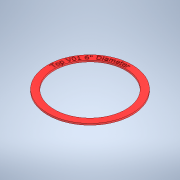
# Autodesk Inventor part: supportRingsForLargeCap
Saved by Autodesk Inventor 2021.1 (Build 251245010, 245A)
## iProperties
Created: 2020-09-25
Part Number: supportRingsForLargeCap
Material: PC/ABS Plastic
Document SubType Name: Modeling
Designer: robst
Density: 0.357273 g/cm^3
Appearance: Light Red
Author: robst
Autodesk Inventor part; units mm, degrees
ref_plane "YZ Plane" through (0, 0, 0) normal (1, 0, 0) x (0, 1, 0)
ref_plane "XZ Plane" through (0, 0, 0) normal (0, 1, 0) x (-1, 0, 0)
ref_plane "XY Plane" through (0, 0, 0) normal (0, 0, 1) x (1, 0, 0)
sketch "Sketch6" plane through (0, 0, 0) normal (0, 0, 1) x (1, 0, 0)
  line L0 (69.85, 0) -> (82.55, 0)
  line L1 (82.55, 0) -> (82.55, 3.175)
  line L2 (82.55, 3.175) -> (69.85, 3.175)
  line L3 (69.85, 3.175) -> (69.85, 0)
  line L4 (0, -0.635) -> (0, 3.81) projected
  point P0 (0, 0)
  dimension "d25" = 12.7
  dimension "d26" = 3.175
  dimension "d27" = 69.85
  constraints: 8 end point, 2 parallel, 1 horizontal, 1 perpendicular
  measures "d25" distance between parallel lines of L1 L3
  measures "d26" distance between parallel lines of L2 L0
  measures "d27" distance of L0.start point (0, 0)
revolve "Revolution3" add sketch "Sketch6" angle 360 about axis through (0, -10, 0) along (0, 1, 0)
sketch "Sketch7" plane through (0, 3.175, 0) normal (0, 1, 0) x (1, 0, 0)
  circle A0 centre (0, 0) radius 76.2 construction
  line L0 (-71.6959, 2.9717) -> (-79.5244, 3.3615)
  line L1 (-79.5244, 3.3615) -> (-79.6728, 0.3827)
  line L2 (-79.6728, 0.3827) -> (-80.7233, 0.435)
  line L3 (-80.7233, 0.435) -> (-80.3678, 7.5727)
  line L4 (-80.3678, 7.5727) -> (-79.3173, 7.5204)
  line L5 (-79.3173, 7.5204) -> (-79.4657, 4.5415)
  line L6 (-79.4657, 4.5415) -> (-71.6372, 4.1517)
  line L7 (-71.6372, 4.1517) -> (-71.6959, 2.9717)
  spline S0 degree 2 poles (-73.8622, 13.8506) (-72.1943, 13.6058) (-70.612, 11.7353) (-70.8087, 10.3953) knots 0 0 0 1 2 2 2
  spline S1 degree 2 poles (-70.8087, 10.3953) (-71.0106, 9.0196) (-73.1164, 7.7194) (-74.7273, 7.9559) knots 0 0 0 1 2 2 2
  spline S2 degree 2 poles (-74.7273, 7.9559) (-76.381, 8.1985) (-77.9743, 10.0925) (-77.7798, 11.4183) knots 0 0 0 1 2 2 2
  spline S3 degree 2 poles (-77.7798, 11.4183) (-77.5831, 12.7583) (-75.523, 14.0943) (-73.8622, 13.8506) knots 0 0 0 1 2 2 2
  spline S4 degree 2 poles (-74.0306, 12.703) (-75.3136, 12.8913) (-76.6981, 12.1406) (-76.8246, 11.2781) knots 0 0 0 1 2 2 2
  spline S5 degree 2 poles (-76.8246, 11.2781) (-76.9512, 10.4157) (-75.8419, 9.2917) (-74.5589, 9.1034) knots 0 0 0 1 2 2 2
  spline S6 degree 2 poles (-74.5589, 9.1034) (-73.3115, 8.9204) (-71.8904, 9.673) (-71.7638, 10.5354) knots 0 0 0 1 2 2 2
  spline S7 degree 2 poles (-71.7638, 10.5354) (-71.6383, 11.3908) (-72.7619, 12.5168) (-74.0306, 12.703) knots 0 0 0 1 2 2 2
  spline S8 degree 2 poles (-72.4154, 20.7565) (-70.7915, 20.3609) (-69.2505, 18.3468) (-69.5387, 17.1639) knots 0 0 0 1 2 2 2
  spline S9 degree 2 poles (-69.5387, 17.1639) (-69.6564, 16.6809) (-70.0611, 15.9935) (-70.3859, 15.6648) knots 0 0 0 1 2 2 2
  line L8 (-70.3859, 15.6648) -> (-67.6701, 15.0032)
  line L9 (-67.6701, 15.0032) -> (-67.9361, 13.9113)
  line L10 (-67.9361, 13.9113) -> (-76.8045, 16.0718)
  line L11 (-76.8045, 16.0718) -> (-76.5385, 17.1638)
  line L12 (-76.5385, 17.1638) -> (-75.8595, 16.9983)
  spline S10 degree 2 poles (-75.8595, 16.9983) (-76.1316, 17.4947) (-76.3794, 18.608) (-76.2379, 19.1889) knots 0 0 0 1 2 2 2
  spline S11 degree 2 poles (-76.2379, 19.1889) (-75.9667, 20.3019) (-73.8993, 21.118) (-72.4154, 20.7565) knots 0 0 0 1 2 2 2
  spline S12 degree 2 poles (-72.564, 19.5989) (-73.6769, 19.8701) (-75.074, 19.4615) (-75.2667, 18.6706) knots 0 0 0 1 2 2 2
  spline S13 degree 2 poles (-75.2667, 18.6706) (-75.3793, 18.2086) (-75.1778, 17.2401) (-74.9496, 16.7767) knots 0 0 0 1 2 2 2
  line L13 (-74.9496, 16.7767) -> (-71.2678, 15.8797)
  spline S14 degree 2 poles (-71.2678, 15.8797) (-70.9608, 16.2572) (-70.6585, 16.8287) (-70.563, 17.2206) knots 0 0 0 1 2 2 2
  spline S15 degree 2 poles (-70.563, 17.2206) (-70.3567, 18.0676) (-71.3741, 19.309) (-72.564, 19.5989) knots 0 0 0 1 2 2 2
  line L14 (-73.177, 34.0889) -> (-66.1232, 27.8719)
  line L15 (-66.1232, 27.8719) -> (-66.6089, 26.6929)
  line L16 (-66.6089, 26.6929) -> (-75.995, 27.2478)
  line L17 (-75.995, 27.2478) -> (-75.5121, 28.4201)
  line L18 (-75.5121, 28.4201) -> (-67.7459, 27.8859)
  line L19 (-67.7459, 27.8859) -> (-73.6353, 32.9764)
  line L20 (-73.6353, 32.9764) -> (-73.177, 34.0889)
  spline S16 degree 2 poles (-65.9446, 38.2865) (-63.8327, 37.1636) (-62.5072, 34.884) (-63.1871, 33.6055) knots 0 0 0 1 2 2 2
  spline S17 degree 2 poles (-63.1871, 33.6055) (-63.877, 32.3079) (-66.5394, 32.1651) (-68.6067, 33.2643) knots 0 0 0 1 2 2 2
  spline S18 degree 2 poles (-68.6067, 33.2643) (-70.7313, 34.3939) (-72.0441, 36.6667) (-71.3609, 37.9516) knots 0 0 0 1 2 2 2
  spline S19 degree 2 poles (-71.3609, 37.9516) (-70.6743, 39.2429) (-67.9928, 39.3755) (-65.9446, 38.2865) knots 0 0 0 1 2 2 2
  spline S20 degree 2 poles (-64.2699, 35.6662) (-64.5767, 36.0252) (-65.7049, 36.7883) (-66.5128, 37.2178) knots 0 0 0 1 2 2 2
  spline S21 degree 2 poles (-66.5128, 37.2178) (-67.3206, 37.6474) (-68.5777, 38.1526) (-69.063, 38.2067) knots 0 0 0 1 2 2 2
  spline S22 degree 2 poles (-69.063, 38.2067) (-69.5483, 38.2607) (-70.256, 37.9272) (-70.4894, 37.4883) knots 0 0 0 1 2 2 2
  spline S23 degree 2 poles (-70.4894, 37.4883) (-70.7228, 37.0493) (-70.6103, 36.2634) (-70.2848, 35.8782) knots 0 0 0 1 2 2 2
  spline S24 degree 2 poles (-70.2848, 35.8782) (-69.9686, 35.5061) (-68.8082, 34.7422) (-68.0385, 34.3329) knots 0 0 0 1 2 2 2
  spline S25 degree 2 poles (-68.0385, 34.3329) (-67.2116, 33.8932) (-66.0507, 33.4065) (-65.5302, 33.3419) knots 0 0 0 1 2 2 2
  spline S26 degree 2 poles (-65.5302, 33.3419) (-65.0419, 33.2781) (-64.302, 33.6109) (-64.0585, 34.0689) knots 0 0 0 1 2 2 2
  spline S27 degree 2 poles (-64.0585, 34.0689) (-63.8285, 34.5014) (-63.941, 35.2874) (-64.2699, 35.6662) knots 0 0 0 1 2 2 2
  line L21 (-58.6672, 41.3818) -> (-61.0498, 37.7579)
  line L22 (-61.0498, 37.7579) -> (-61.8083, 38.2566)
  line L23 (-61.8083, 38.2566) -> (-60.9217, 39.605)
  line L24 (-60.9217, 39.605) -> (-65.9001, 42.878)
  line L25 (-65.9001, 42.878) -> (-66.7866, 41.5296)
  line L26 (-66.7866, 41.5296) -> (-67.4668, 41.9768)
  spline S28 degree 2 poles (-67.4668, 41.9768) (-66.9642, 42.7413) (-66.9227, 43.7486) (-67.493, 44.1926) knots 0 0 0 1 2 2 2
  line L27 (-67.493, 44.1926) -> (-66.9864, 44.9631)
  line L28 (-66.9864, 44.9631) -> (-60.2925, 40.5621)
  line L29 (-60.2925, 40.5621) -> (-59.4257, 41.8804)
  line L30 (-59.4257, 41.8804) -> (-58.6672, 41.3818)
  spline S29 degree 2 poles (-53.7813, 51.8344) (-53.2703, 51.3792) (-52.7061, 50.2688) (-52.6695, 49.7249) knots 0 0 0 1 2 2 2
  spline S30 degree 2 poles (-52.6695, 49.7249) (-52.6265, 49.1559) (-52.9704, 48.1308) (-53.3681, 47.6843) knots 0 0 0 1 2 2 2
  spline S31 degree 2 poles (-53.3681, 47.6843) (-53.7658, 47.2378) (-54.7236, 46.7692) (-55.274, 46.7578) knots 0 0 0 1 2 2 2
  spline S32 degree 2 poles (-55.274, 46.7578) (-55.9411, 46.7346) (-57.4965, 47.4254) (-58.3787, 48.2113) knots 0 0 0 1 2 2 2
  spline S33 degree 2 poles (-58.3787, 48.2113) (-59.2448, 48.9828) (-60.3218, 50.579) (-60.5076, 51.4102) knots 0 0 0 1 2 2 2
  spline S34 degree 2 poles (-60.5076, 51.4102) (-60.6922, 52.221) (-60.2411, 53.8646) (-59.5751, 54.6123) knots 0 0 0 1 2 2 2
  spline S35 degree 2 poles (-59.5751, 54.6123) (-59.3786, 54.8329) (-58.9905, 55.1819) (-58.8128, 55.284) knots 0 0 0 1 2 2 2
  line L31 (-58.8128, 55.284) -> (-57.9574, 54.5221)
  line L32 (-57.9574, 54.5221) -> (-57.991, 54.4844)
  spline S36 degree 2 poles (-57.991, 54.4844) (-58.1657, 54.4182) (-58.6812, 54.067) (-58.9112, 53.8088) knots 0 0 0 1 2 2 2
  spline S37 degree 2 poles (-58.9112, 53.8088) (-59.6492, 52.9803) (-59.4359, 50.9669) (-58.4248, 49.8925) knots 0 0 0 1 2 2 2
  spline S38 degree 2 poles (-58.4248, 49.8925) (-58.3626, 50.4064) (-58.0105, 51.2891) (-57.6559, 51.6871) knots 0 0 0 1 2 2 2
  spline S39 degree 2 poles (-57.6559, 51.6871) (-57.3109, 52.0744) (-56.6374, 52.5165) (-56.1179, 52.623) knots 0 0 0 1 2 2 2
  spline S40 degree 2 poles (-56.1179, 52.623) (-55.5177, 52.7444) (-54.3515, 52.3423) (-53.7813, 51.8344) knots 0 0 0 1 2 2 2
  spline S41 degree 2 poles (-54.5487, 50.8971) (-54.9575, 51.2613) (-55.7033, 51.5397) (-56.1078, 51.4755) knots 0 0 0 1 2 2 2
  spline S42 degree 2 poles (-56.1078, 51.4755) (-56.4058, 51.4226) (-56.8902, 51.0629) (-57.0962, 50.8316) knots 0 0 0 1 2 2 2
  spline S43 degree 2 poles (-57.0962, 50.8316) (-57.3742, 50.5196) (-57.7082, 49.7655) (-57.7846, 49.3223) knots 0 0 0 1 2 2 2
  spline S44 degree 2 poles (-57.7846, 49.3223) (-57.6926, 49.2306) (-57.5193, 49.057) (-57.3794, 48.9324) knots 0 0 0 1 2 2 2
  spline S45 degree 2 poles (-57.3794, 48.9324) (-56.6909, 48.319) (-55.6067, 47.8356) (-55.204, 47.8436) knots 0 0 0 1 2 2 2
  spline S46 degree 2 poles (-55.204, 47.8436) (-54.8265, 47.845) (-54.2956, 48.1053) (-54.0895, 48.3366) knots 0 0 0 1 2 2 2
  spline S47 degree 2 poles (-54.0895, 48.3366) (-53.6103, 48.8745) (-53.7848, 50.2167) (-54.5487, 50.8971) knots 0 0 0 1 2 2 2
  line L33 (-54.6918, 59.8301) -> (-52.4909, 57.1504)
  line L34 (-52.4909, 57.1504) -> (-53.0587, 56.608)
  line L35 (-53.0587, 56.608) -> (-55.6347, 58.9294)
  line L36 (-55.6347, 58.9294) -> (-54.6918, 59.8301)
  line L37 (-56.3172, 58.2776) -> (-54.1163, 55.5978)
  line L38 (-54.1163, 55.5978) -> (-54.6841, 55.0555)
  line L39 (-54.6841, 55.0555) -> (-57.2601, 57.3769)
  line L40 (-57.2601, 57.3769) -> (-56.3172, 58.2776)
  spline S48 degree 2 poles (-41.0388, 64.3065) (-40.334, 63.3137) (-40.0044, 61.1446) (-40.363, 60.2185) knots 0 0 0 1 2 2 2
  spline S49 degree 2 poles (-40.363, 60.2185) (-40.6691, 59.4799) (-41.636, 58.44) (-42.5172, 57.8144) knots 0 0 0 1 2 2 2
  line L41 (-42.5172, 57.8144) -> (-44.1855, 56.63)
  line L42 (-44.1855, 56.63) -> (-49.3319, 63.8789)
  line L43 (-49.3319, 63.8789) -> (-47.6813, 65.0508)
  spline S50 degree 2 poles (-47.6813, 65.0508) (-46.6591, 65.7765) (-45.2791, 66.2968) (-44.6761, 66.3185) knots 0 0 0 1 2 2 2
  spline S51 degree 2 poles (-44.6761, 66.3185) (-43.6476, 66.3507) (-41.7895, 65.3639) (-41.0388, 64.3065) knots 0 0 0 1 2 2 2
  spline S52 degree 2 poles (-42.0517, 63.6051) (-42.6439, 64.4392) (-44.0344, 65.2279) (-44.8184, 65.1749) knots 0 0 0 1 2 2 2
  spline S53 degree 2 poles (-44.8184, 65.1749) (-45.3688, 65.1287) (-46.39, 64.7129) (-47.042, 64.25) knots 0 0 0 1 2 2 2
  line L44 (-47.042, 64.25) -> (-47.7763, 63.7287)
  line L45 (-47.7763, 63.7287) -> (-43.8143, 58.1481)
  line L46 (-43.8143, 58.1481) -> (-43.08, 58.6694)
  spline S54 degree 2 poles (-43.08, 58.6694) (-42.4397, 59.124) (-41.6164, 60.0178) (-41.4189, 60.5733) knots 0 0 0 1 2 2 2
  spline S55 degree 2 poles (-41.4189, 60.5733) (-41.1556, 61.2726) (-41.4511, 62.7592) (-42.0517, 63.6051) knots 0 0 0 1 2 2 2
  line L47 (-36.4216, 61.8269) -> (-37.3855, 61.2489)
  line L48 (-37.3855, 61.2489) -> (-40.8164, 66.9701)
  line L49 (-40.8164, 66.9701) -> (-39.8526, 67.5481)
  line L50 (-39.8526, 67.5481) -> (-36.4216, 61.8269)
  line L51 (-40.3552, 68.5403) -> (-41.4488, 67.8845)
  line L52 (-41.4488, 67.8845) -> (-42.049, 68.8854)
  line L53 (-42.049, 68.8854) -> (-40.9554, 69.5412)
  line L54 (-40.9554, 69.5412) -> (-40.3552, 68.5403)
  spline S56 degree 2 poles (-32.0297, 65.0111) (-32.1051, 64.8587) (-32.3499, 64.3273) (-32.4925, 64.1322) knots 0 0 0 1 2 2 2
  spline S57 degree 2 poles (-32.4925, 64.1322) (-32.6824, 63.856) (-33.0995, 63.4545) (-33.5477, 63.2234) knots 0 0 0 1 2 2 2
  spline S58 degree 2 poles (-33.5477, 63.2234) (-33.9127, 63.0352) (-34.7142, 62.9706) (-35.0927, 63.0915) knots 0 0 0 1 2 2 2
  spline S59 degree 2 poles (-35.0927, 63.0915) (-35.4551, 63.2127) (-36.113, 63.7813) (-36.3176, 64.1783) knots 0 0 0 1 2 2 2
  spline S60 degree 2 poles (-36.3176, 64.1783) (-36.6346, 64.793) (-36.5649, 65.9313) (-36.1301, 66.4715) knots 0 0 0 1 2 2 2
  spline S61 degree 2 poles (-36.1301, 66.4715) (-35.7495, 66.9596) (-34.4811, 67.8323) (-33.7166, 68.2832) knots 0 0 0 1 2 2 2
  line L55 (-33.7166, 68.2832) -> (-33.8157, 68.4753)
  spline S62 degree 2 poles (-33.8157, 68.4753) (-33.994, 68.8211) (-34.4264, 69.1412) (-34.6813, 69.1638) knots 0 0 0 1 2 2 2
  spline S63 degree 2 poles (-34.6813, 69.1638) (-34.9361, 69.1864) (-35.5264, 68.9793) (-35.8209, 68.8275) knots 0 0 0 1 2 2 2
  spline S64 degree 2 poles (-35.8209, 68.8275) (-36.1667, 68.6492) (-36.996, 67.9623) (-37.3611, 67.5228) knots 0 0 0 1 2 2 2
  line L56 (-37.3611, 67.5228) -> (-37.4187, 67.4931)
  line L57 (-37.4187, 67.4931) -> (-37.9436, 68.5112)
  spline S65 degree 2 poles (-37.9436, 68.5112) (-37.7079, 68.73) (-36.776, 69.4536) (-36.2701, 69.7144) knots 0 0 0 1 2 2 2
  spline S66 degree 2 poles (-36.2701, 69.7144) (-35.6554, 70.0314) (-34.7175, 70.2717) (-34.2558, 70.1937) knots 0 0 0 1 2 2 2
  spline S67 degree 2 poles (-34.2558, 70.1937) (-33.8038, 70.1187) (-33.0842, 69.509) (-32.797, 68.9519) knots 0 0 0 1 2 2 2
  line L58 (-32.797, 68.9519) -> (-30.7073, 64.8986)
  line L59 (-30.7073, 64.8986) -> (-31.7062, 64.3836)
  line L60 (-31.7062, 64.3836) -> (-32.0297, 65.0111)
  line L61 (-32.4589, 65.8435) -> (-33.3073, 67.4892)
  spline S68 degree 2 poles (-33.3073, 67.4892) (-33.6494, 67.2723) (-34.6754, 66.6055) (-34.962, 66.3281) knots 0 0 0 1 2 2 2
  spline S69 degree 2 poles (-34.962, 66.3281) (-35.2962, 66.0018) (-35.5541, 65.2285) (-35.323, 64.7803) knots 0 0 0 1 2 2 2
  spline S70 degree 2 poles (-35.323, 64.7803) (-35.0589, 64.268) (-34.2152, 64.0465) (-33.6645, 64.3304) knots 0 0 0 1 2 2 2
  spline S71 degree 2 poles (-33.6645, 64.3304) (-33.1971, 64.5714) (-32.6367, 65.3709) (-32.4589, 65.8435) knots 0 0 0 1 2 2 2
  line L62 (-22.2335, 68.3007) -> (-23.5934, 71.9148)
  spline S72 degree 2 poles (-23.5934, 71.9148) (-23.7558, 72.3463) (-24.0998, 73.0559) (-24.2838, 73.2175) knots 0 0 0 1 2 2 2
  spline S73 degree 2 poles (-24.2838, 73.2175) (-24.4754, 73.3995) (-24.9679, 73.4605) (-25.3252, 73.326) knots 0 0 0 1 2 2 2
  spline S74 degree 2 poles (-25.3252, 73.326) (-25.6489, 73.2042) (-26.2409, 72.5273) (-26.4899, 72.0025) knots 0 0 0 1 2 2 2
  spline S75 degree 2 poles (-26.4899, 72.0025) (-26.4476, 71.9107) (-26.3352, 71.6528) (-26.2692, 71.4775) knots 0 0 0 1 2 2 2
  line L63 (-26.2692, 71.4775) -> (-24.7215, 67.3645)
  line L64 (-24.7215, 67.3645) -> (-25.7734, 66.9687)
  line L65 (-25.7734, 66.9687) -> (-27.1333, 70.5827)
  spline S76 degree 2 poles (-27.1333, 70.5827) (-27.2957, 71.0142) (-27.6397, 71.7238) (-27.8237, 71.8855) knots 0 0 0 1 2 2 2
  spline S77 degree 2 poles (-27.8237, 71.8855) (-28.0153, 72.0674) (-28.5078, 72.1284) (-28.8651, 71.9939) knots 0 0 0 1 2 2 2
  spline S78 degree 2 poles (-28.8651, 71.9939) (-29.2023, 71.8671) (-29.7909, 71.1607) (-30.0172, 70.6983) knots 0 0 0 1 2 2 2
  line L66 (-30.0172, 70.6983) -> (-28.2614, 66.0324)
  line L67 (-28.2614, 66.0324) -> (-29.3133, 65.6366)
  line L68 (-29.3133, 65.6366) -> (-31.6627, 71.8803)
  line L69 (-31.6627, 71.8803) -> (-30.6109, 72.2761)
  line L70 (-30.6109, 72.2761) -> (-30.3521, 71.5884)
  spline S79 degree 2 poles (-30.3521, 71.5884) (-30.0955, 72.1544) (-29.4564, 72.9107) (-28.9709, 73.0933) knots 0 0 0 1 2 2 2
  spline S80 degree 2 poles (-28.9709, 73.0933) (-28.418, 73.3014) (-27.3714, 73.1179) (-26.9333, 72.6285) knots 0 0 0 1 2 2 2
  spline S81 degree 2 poles (-26.9333, 72.6285) (-26.655, 73.3413) (-25.957, 74.2275) (-25.4311, 74.4254) knots 0 0 0 1 2 2 2
  spline S82 degree 2 poles (-25.4311, 74.4254) (-25.0265, 74.5776) (-24.2718, 74.5768) (-23.9225, 74.3849) knots 0 0 0 1 2 2 2
  spline S83 degree 2 poles (-23.9225, 74.3849) (-23.5665, 74.1956) (-22.9704, 73.4501) (-22.7293, 72.8095) knots 0 0 0 1 2 2 2
  line L71 (-22.7293, 72.8095) -> (-21.1816, 68.6965)
  line L72 (-21.1816, 68.6965) -> (-22.2335, 68.3007)
  spline S84 degree 2 poles (-16.7982, 69.6072) (-18.3503, 69.2213) (-20.489, 70.538) (-20.8888, 72.146) knots 0 0 0 1 2 2 2
  spline S85 degree 2 poles (-20.8888, 72.146) (-21.2817, 73.726) (-20.0906, 76.0117) (-18.7552, 76.3437) knots 0 0 0 1 2 2 2
  spline S86 degree 2 poles (-18.7552, 76.3437) (-18.154, 76.4932) (-17.1372, 76.3748) (-16.7025, 76.0894) knots 0 0 0 1 2 2 2
  spline S87 degree 2 poles (-16.7025, 76.0894) (-16.2608, 75.8058) (-15.6243, 74.8283) (-15.4313, 74.0522) knots 0 0 0 1 2 2 2
  line L73 (-15.4313, 74.0522) -> (-15.2836, 73.458)
  line L74 (-15.2836, 73.458) -> (-19.765, 72.3437)
  spline S88 degree 2 poles (-19.765, 72.3437) (-19.4852, 71.2181) (-18.0553, 70.3042) (-17.0486, 70.5545) knots 0 0 0 1 2 2 2
  spline S89 degree 2 poles (-17.0486, 70.5545) (-16.692, 70.6432) (-16.0399, 70.976) (-15.7915, 71.1714) knots 0 0 0 1 2 2 2
  spline S90 degree 2 poles (-15.7915, 71.1714) (-15.5326, 71.3843) (-15.188, 71.7298) (-15.0829, 71.8747) knots 0 0 0 1 2 2 2
  line L75 (-15.0829, 71.8747) -> (-15.02, 71.8903)
  line L76 (-15.02, 71.8903) -> (-14.7245, 70.7018)
  spline S91 degree 2 poles (-14.7245, 70.7018) (-14.8941, 70.5779) (-15.4118, 70.2117) (-15.6199, 70.0931) knots 0 0 0 1 2 2 2
  spline S92 degree 2 poles (-15.6199, 70.0931) (-15.9119, 69.924) (-16.4067, 69.7045) (-16.7982, 69.6072) knots 0 0 0 1 2 2 2
  spline S93 degree 2 poles (-16.5531, 74.0257) (-16.6766, 74.4627) (-17.0183, 75.0607) (-17.247, 75.234) knots 0 0 0 1 2 2 2
  spline S94 degree 2 poles (-17.247, 75.234) (-17.4966, 75.4317) (-18.1552, 75.5427) (-18.5956, 75.4332) knots 0 0 0 1 2 2 2
  spline S95 degree 2 poles (-18.5956, 75.4332) (-19.0291, 75.3254) (-19.573, 74.9155) (-19.7621, 74.6012) knots 0 0 0 1 2 2 2
  spline S96 degree 2 poles (-19.7621, 74.6012) (-19.9425, 74.2817) (-20.0395, 73.5969) (-19.9719, 73.1757) knots 0 0 0 1 2 2 2
  line L77 (-19.9719, 73.1757) -> (-16.5531, 74.0257)
  spline S97 degree 2 poles (-11.3712, 70.7213) (-12.2729, 70.5661) (-13.4653, 71.4209) (-13.6571, 72.5356) knots 0 0 0 1 2 2 2
  line L78 (-13.6571, 72.5356) -> (-14.2838, 76.1779)
  line L79 (-14.2838, 76.1779) -> (-15.0293, 76.0496)
  line L80 (-15.0293, 76.0496) -> (-15.1869, 76.9655)
  line L81 (-15.1869, 76.9655) -> (-14.4414, 77.0937)
  line L82 (-14.4414, 77.0937) -> (-14.7663, 78.9823)
  line L83 (-14.7663, 78.9823) -> (-13.6587, 79.1729)
  line L84 (-13.6587, 79.1729) -> (-13.3338, 77.2843)
  line L85 (-13.3338, 77.2843) -> (-11.2961, 77.6349)
  line L86 (-11.2961, 77.6349) -> (-11.1385, 76.719)
  line L87 (-11.1385, 76.719) -> (-13.1762, 76.3684)
  line L88 (-13.1762, 76.3684) -> (-12.6375, 73.2374)
  spline S98 degree 2 poles (-12.6375, 73.2374) (-12.552, 72.7404) (-12.4224, 72.1998) (-12.2614, 71.9863) knots 0 0 0 1 2 2 2
  spline S99 degree 2 poles (-12.2614, 71.9863) (-12.1266, 71.7975) (-11.6439, 71.6685) (-11.2605, 71.7345) knots 0 0 0 1 2 2 2
  spline S100 degree 2 poles (-11.2605, 71.7345) (-10.9907, 71.7809) (-10.5147, 72.031) (-10.4096, 72.1002) knots 0 0 0 1 2 2 2
  line L89 (-10.4096, 72.1002) -> (-10.3457, 72.1112)
  line L90 (-10.3457, 72.1112) -> (-10.1747, 71.1172)
  spline S101 degree 2 poles (-10.1747, 71.1172) (-10.4725, 70.9783) (-11.0943, 70.7689) (-11.3712, 70.7213) knots 0 0 0 1 2 2 2
  spline S102 degree 2 poles (-6.4494, 71.3144) (-8.0413, 71.1593) (-9.9647, 72.7744) (-10.1253, 74.4235) knots 0 0 0 1 2 2 2
  spline S103 degree 2 poles (-10.1253, 74.4235) (-10.2831, 76.044) (-8.7709, 78.1312) (-7.4014, 78.2645) knots 0 0 0 1 2 2 2
  spline S104 degree 2 poles (-7.4014, 78.2645) (-6.7847, 78.3246) (-5.7962, 78.0589) (-5.4078, 77.7131) knots 0 0 0 1 2 2 2
  spline S105 degree 2 poles (-5.4078, 77.7131) (-5.0123, 77.368) (-4.5254, 76.308) (-4.4479, 75.5121) knots 0 0 0 1 2 2 2
  line L91 (-4.4479, 75.5121) -> (-4.3885, 74.9026)
  line L92 (-4.3885, 74.9026) -> (-8.9847, 74.455)
  spline S106 degree 2 poles (-8.9847, 74.455) (-8.8723, 73.3006) (-7.5913, 72.1876) (-6.5588, 72.2881) knots 0 0 0 1 2 2 2
  spline S107 degree 2 poles (-6.5588, 72.2881) (-6.1931, 72.3237) (-5.4993, 72.5578) (-5.225, 72.7148) knots 0 0 0 1 2 2 2
  spline S108 degree 2 poles (-5.225, 72.7148) (-4.9378, 72.8875) (-4.5464, 73.179) (-4.4213, 73.307) knots 0 0 0 1 2 2 2
  line L93 (-4.4213, 73.307) -> (-4.3568, 73.3133)
  line L94 (-4.3568, 73.3133) -> (-4.2381, 72.0943)
  spline S109 degree 2 poles (-4.2381, 72.0943) (-4.424, 71.9966) (-4.9896, 71.7099) (-5.2128, 71.623) knots 0 0 0 1 2 2 2
  spline S110 degree 2 poles (-5.2128, 71.623) (-5.5264, 71.4984) (-6.0479, 71.3535) (-6.4494, 71.3144) knots 0 0 0 1 2 2 2
  spline S111 degree 2 poles (-5.5615, 75.6497) (-5.6199, 76.1001) (-5.8705, 76.7416) (-6.0714, 76.9464) knots 0 0 0 1 2 2 2
  spline S112 degree 2 poles (-6.0714, 76.9464) (-6.2895, 77.1785) (-6.9248, 77.3844) (-7.3765, 77.3404) knots 0 0 0 1 2 2 2
  spline S113 degree 2 poles (-7.3765, 77.3404) (-7.8211, 77.2972) (-8.4191, 76.9711) (-8.652, 76.6878) knots 0 0 0 1 2 2 2
  spline S114 degree 2 poles (-8.652, 76.6878) (-8.8772, 76.3981) (-9.0732, 75.7348) (-9.0678, 75.3083) knots 0 0 0 1 2 2 2
  line L95 (-9.0678, 75.3083) -> (-5.5615, 75.6497)
  line L96 (0.4806, 77.2513) -> (0.423, 77.2501)
  spline S115 degree 2 poles (0.423, 77.2501) (0.2926, 77.2833) (0.0114, 77.2917) (-0.1831, 77.2875) knots 0 0 0 1 2 2 2
  spline S116 degree 2 poles (-0.1831, 77.2875) (-0.6368, 77.2777) (-1.5214, 76.8623) (-1.9164, 76.4646) knots 0 0 0 1 2 2 2
  line L97 (-1.9164, 76.4646) -> (-1.8143, 71.7326)
  line L98 (-1.8143, 71.7326) -> (-2.9379, 71.7083)
  line L99 (-2.9379, 71.7083) -> (-3.0818, 78.3779)
  line L100 (-3.0818, 78.3779) -> (-1.9582, 78.4021)
  line L101 (-1.9582, 78.4021) -> (-1.9367, 77.4082)
  spline S117 degree 2 poles (-1.9367, 77.4082) (-1.3363, 77.9688) (-0.4312, 78.435) (0.0009, 78.4444) knots 0 0 0 1 2 2 2
  spline S118 degree 2 poles (0.0009, 78.4444) (0.1738, 78.4481) (0.347, 78.4374) (0.4555, 78.4182) knots 0 0 0 1 2 2 2
  line L102 (0.4555, 78.4182) -> (0.4806, 77.2513)
  dimension "d29" = 152.4
  constraints: 1 centre point, 1 coincident, 1 other
  measures "d29" diameter of A0
extrude "Extrusion3" cut sketch "Sketch7" against normal blind 1.27
equation "\"d25\" = outsideRingWidth"
equation "\"d26\" = ringHeight"
equation "\"d27\" = outsideRingInnerEdge"
equation "\"thickness\" = 6.35"
equation "\"outsideRingDiameter\" = 152.4"
equation "\"textRingDiameter\" = 76.2"
equation "\"textRingDepth\" = 1.27"
equation "\"outsideRingRadius\" = 0.5 * outsideRingDiameter"
equation "\"outsideRingWidth\" = 12.7"
equation "\"ringHeight\" = 3.175"
equation "\"outsideRingInnerEdge\" = outsideRingRadius - 0.5 * outsideRingWidth"
body "Solid3"
